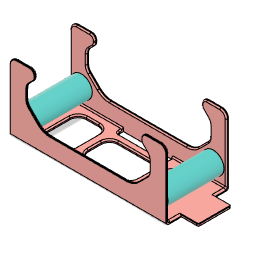
Spool Holder + Rollers D6 (Autodesk Fusion 360 design; units mm, degrees)
Autodesk Fusion 360 part; units mm, degrees
note: some values were not read from the file. Chosen so that the rebuilt part matches the saved one: which bodies a step acts on. Set by a fixed rule: which sketch regions a step uses.
sketch "Sketch1" plane through (0, 0, 0) normal (0, 1, 0) x (1, 0, 0) in component "Base"
  line L0 (-22.8106, -31.0965) -> (-3.5106, -30.609)
  line L1 (3.8, -23.1114) -> (3.8, 23.119)
  line L2 (40.5, -22.1842) -> (40.5, 22.1918)
  line L3 (13.7394, -30.1732) -> (33.1894, -29.6818)
  line L4 (13.7394, 30.1808) -> (33.1894, 29.6894)
  line L5 (-22.8106, 31.1041) -> (-3.5106, 30.6166)
  line L6 (-30.5, -23.5989) -> (-30.5, 23.6065)
  line L7 (6.05, -22.6756) -> (6.05, 22.6832)
  line L8 (95, 35) -> (-95, 35)
  line L9 (-95, 35) -> (-95, -35)
  line L10 (-95, -35) -> (95, -35)
  line L11 (95, -35) -> (95, 35)
  line L12 (95, 35) -> (-95, -35) construction
  line L13 (-95, 35) -> (95, -35) construction
  line L14 (-95, -35) -> (95, -35)
  line L15 (95, -35) -> (95, -38)
  line L16 (95, -38) -> (-95, -38)
  line L17 (-95, -38) -> (-95, -35)
  line L18 (-95, 35) -> (95, 35)
  line L19 (95, 35) -> (95, 38)
  line L20 (95, 38) -> (-95, 38)
  line L21 (-95, 38) -> (-95, 35)
  line L22 (0, -35) -> (0, 35) construction
  line L23 (-75, -25) -> (-40, -25)
  line L24 (-40, -25) -> (-40, 25)
  line L25 (-40, 25) -> (-75, 25)
  line L26 (-75, 25) -> (-75, -25)
  line L27 (40, -25) -> (75, -25)
  line L28 (75, -25) -> (75, 25)
  line L29 (75, 25) -> (40, 25)
  line L30 (40, 25) -> (40, -25)
  line L31 (-30, 18) -> (30, 18)
  line L32 (30, 18) -> (30, -18)
  line L33 (30, -18) -> (-30, -18)
  line L34 (-30, -18) -> (-30, 18)
  line L35 (-30, 38) -> (-30, 27)
  line L36 (30, 38) -> (30, 27)
  line L37 (-30, -27) -> (-30, -38)
  line L38 (30, -27) -> (30, -38)
  line L39 (-30, -27) -> (30, -27)
  line L40 (-30, 27) -> (30, 27)
  line L41 (95, 20) -> (114, 20)
  line L42 (116, 18) -> (116, -18)
  line L43 (114, -20) -> (95, -20)
  arc A0 (116, 18) -> (114, 20) centre (114, 18) ccw
  arc A1 (114, -20) -> (116, -18) centre (114, -18) ccw
  point P0 (-42.5, 38.6038)
  point P1 (-42.5, 36.7032)
  point P2 (52.5, 36.2038)
  point P3 (52.5, 34.3032)
  point P4 (52.5, -36.1962)
  point P5 (52.5, -34.2956)
  point P6 (-42.5, -36.6956)
  point P7 (-42.5, -38.5962)
  point P8 (52.5, 36.2038)
  point P9 (52.5, 34.3032)
  point P10 (52.5, -34.2956)
  point P11 (52.5, -36.1962)
  point P12 (-42.5, -38.5962)
  point P13 (-42.5, -36.6956)
  point P14 (-42.5, 36.7032)
  point P15 (-42.5, 38.6038)
  point P16 (0, -35)
  point P17 (0, 35)
  point P18 (0, 18)
  point P19 (-95, 0)
  point P20 (95, 0)
  point P21 (116, 20)
  dimension "d1" = 70
  dimension "d2" = 190
  dimension "d3" = 3
  dimension "d4" = 20
  dimension "d5" = 10
  dimension "d6" = 10
  dimension "d9" = 10
  dimension "d10" = 10
  dimension "d11" = 20
  dimension "d91" = 10
  dimension "d92" = 10
  dimension "d93" = 35
  dimension "d94" = 35
  dimension "d95" = 30
  dimension "d96" = 30
  dimension "d100" = 8
  dimension "d102" = 18
  dimension "d103" = 18
  dimension "d104" = 60
  dimension "d137" = 20
  dimension "d138" = 20
  dimension "d139" = 21
  dimension "d140" = 2
  dimension "d141" = 2
  constraint coincident P8 P2
  constraint coincident P9 P3
  constraint coincident P10 P5
  constraint coincident P11 P4
  constraint coincident P14 P1
  constraint coincident P15 P0
  constraint coincident P13 P6
  constraint coincident P12 P7
  constraint horizontal L8
  constraint perpendicular L8 L9
  constraint parallel L8 L10
  constraint parallel L9 L11
  constraint coincident L12 origin
  constraint coincident L13 origin
  constraint horizontal L14
  constraint vertical L15
  constraint horizontal L16
  constraint vertical L17
  constraint horizontal L18
  constraint vertical L19
  constraint horizontal L20
  constraint vertical L21
  constraint coincident L8.end L9.start
  constraint coincident L8.start L11.end
  constraint coincident L9.end L10.start
  constraint coincident L10.end L11.start
  constraint equal L17 L21
  constraint midpoint L14 P16
  constraint midpoint L8 P17
  constraint coincident P16 L22.start
  constraint coincident P17 L22.end
  constraint horizontal L23
  constraint vertical L24
  constraint horizontal L25
  constraint vertical L26
  constraint horizontal L27
  constraint vertical L28
  constraint horizontal L29
  constraint vertical L30
  constraint horizontal L31
  constraint vertical L32
  constraint horizontal L33
  constraint vertical L34
  constraint midpoint L31 P18
  constraint coincident L22 P18
  constraint vertical L35
  constraint vertical L36
  constraint perpendicular L16 L37
  constraint perpendicular L14 L38
  constraint coincident L20 L35.start
  constraint coincident L20 L36.start
  constraint coincident L16 L38.end
  constraint coincident L16 L37.end
  constraint horizontal L39
  constraint perpendicular L7 L40
  constraint coincident L37.start L39.start
  constraint coincident L38.start L39.end
  constraint coincident L35.end L40.start
  constraint coincident L36.end L40.end
  constraint collinear L35 L37
  constraint collinear L36 L38
  constraint equal L36 L38
  constraint midpoint L9 P19
  constraint midpoint L11 P20
  constraint horizontal L41
  constraint horizontal L43
  constraint vertical L42
  constraint coincident L11 L41.start
  constraint coincident L11 L43.end
  constraint coincident P21 L42
  constraint coincident P21 L41
  constraint tangent L42 A0
  constraint tangent L41 A0
  constraint tangent L42 A1
  constraint tangent L43 A1
  measures "d1" distance of L8.end L9.end
  measures "d2" distance of L8.start L8.end
  measures "d3" distance of L9.end L16.end
  measures "d4" distance of L9 L26
  measures "d5" distance of L14 L23
  measures "d6" distance of L8 L25
  measures "d9" distance of L18 L29
  measures "d10" distance of L10 L27
  measures "d11" distance of L11 L28
  measures "d91" distance of L24 L34
  measures "d92" distance of L30 L32
  measures "d93" distance of L24.end L25.end
  measures "d94" distance of L28 L30
  measures "d95" distance of P17 L35
  measures "d96" distance of P17 L36
  measures "d100" distance of L8 L40
  measures "d102" distance of origin L31
  measures "d103" distance of origin L33
  measures "d104" distance of L32 L34
  measures "d137" distance of P20 L43.end
  measures "d138" distance of P20 L41.start
  measures "d139" distance of L41.start P21
  measures "d140" radius of A0
  measures "d141" radius of A1
extrude "Extrude1" add sketch "Sketch1" along normal blind 100 contours L8 L18 L19 L20 L36 | L8 L18 L20 L35 L36 | L8 L18 L20 L21 L35 makes body 1 in component "Base"
extrude "Extrude2" add sketch "Sketch1" along normal blind 100 separate body contours L10 L14 L15 L16 L38 | L10 L14 L16 L17 L37 | L10 L14 L16 L37 L38 makes body 2 in component "Base"
extrude "Extrude3" add sketch "Sketch1" against normal blind 3 contours L8 L9 L10 L11 L14 L18 L35 L36 L37 L38 L39 L40 | L8 L18 L19 L20 L36 | L8 L18 L20 L35 L36 | L11 L41 L42 L43 A0 A1 | L8 L18 L20 L21 L35 | L10 L14 L15 L16 L38 | L10 L14 L16 L17 L37 | L10 L14 L16 L37 L38 bodies 1 2 in component "Base"
sketch "Sketch2" plane through (0, 0, -35) normal (0, 0, 1) x (1, 0, 0) in component "Base"
  circle A0 centre (-80, 20) radius 3.9
  circle A1 centre (-80, 20) radius 6
  line L0 (95, 0) -> (95, 100)
  line L1 (95, 100) -> (-95, 100)
  line L2 (-95, 100) -> (-95, 0)
  line L3 (-95, 0) -> (-30, 0)
  line L4 (0, 100) -> (0, 0) construction
  line L5 (-30, 0) -> (-30, -3)
  line L6 (-30, -3) -> (30, -3)
  line L7 (30, -3) -> (30, 0)
  line L8 (30, 0) -> (95, 0)
  line L9 (1.75, 0) -> (22.5, 0)
  line L10 (-55, 20) -> (55, 20)
  line L11 (55, 20) -> (75, 40)
  line L12 (-75, 40) -> (-55, 20)
  line L13 (65, 80) -> (95, 80)
  line L14 (65, 80) -> (65, 70)
  line L15 (65, 70) -> (75, 60)
  line L16 (75, 60) -> (75, 40)
  line L17 (-75, 40) -> (-75, 60)
  line L18 (-75, 60) -> (-65, 70)
  line L19 (-65, 70) -> (-65, 80)
  line L20 (-65, 80) -> (-95, 80)
  point P0 (-80, 20)
  point P1 (0, 20)
  point P2 (0, 80)
  dimension "d29" = 80
  dimension "d30" = 20
  dimension "d31" = 7.8
  dimension "d32" = 12
  dimension "d176" = 135
  dimension "d177" = 135
  dimension "d181" = 20
  dimension "d185" = 20
  dimension "d204" = 20
  dimension "d205" = 135
  dimension "d206" = 30
  dimension "d207" = 10
  dimension "d208" = 80
  dimension "d209" = 135
  constraint coincident P0 A0.centre
  constraint coincident L1 L4.start
  constraint coincident L4.end origin
  constraint horizontal L10
  constraint equal L11 L12
  constraint midpoint L10 P1
  constraint coincident L4 P1
  constraint coincident L4 P2
  constraint perpendicular L4 L9
  constraint horizontal L13
  constraint coincident L0 L13.end
  constraint vertical L16
  constraint coincident L13.start L14.start
  constraint vertical L14
  constraint coincident L2 L20.end
  constraint horizontal L20
  constraint vertical L19
  constraint vertical L17
  constraint equal L13 L20
  constraint equal L14 L19
  constraint equal L16 L17
  measures "d29" horizontal distance of P0 L4.end
  measures "d30" vertical distance of P0 L4.end
  measures "d31" diameter of A0
  measures "d32" diameter of A1
  measures "d176" angle of L10 L12
  measures "d177" angle of L10 L11
  measures "d181" distance of L8 L10
  measures "d185" vertical distance of L10.start L12.start
  measures "d204" distance of L0 L16
  measures "d205" angle of L14 L15
  measures "d206" distance of L13.start L13.end
  measures "d207" distance of L13.start L14.end
  measures "d208" distance of L8 L13
  measures "d209" angle of L18 L19
extrude "Extrude4" add sketch "Sketch2" along normal blind 6 separate body contours A0 makes body 3 in component "Base"
extrude "Extrude5" add sketch "Sketch2" along normal blind 2 contours A1 bodies 3 in component "Base"
extrude "Extrude9" cut sketch "Sketch2" along normal through all and the other way through all contours L0 L1 L2 L10 L11 L12 L13 L14 L15 L16 L17 L18 L19 L20 bodies 1 in component "Base"
sketch "Sketch3" plane through (0, 0, -29) normal (0, 0, 1) x (1, 0, 0) in component "Base"
  circle A0 centre (-80, 20) radius 3.9
  line L0 (-83.9, 20) -> (-76.1, 20)
  circle A1 centre (-80, 20) radius 3.9
  point P0 (-80, 20)
  point P1 (-80, 20)
  dimension "d37" = 7.8
  constraint coincident P0 A0.centre
  constraint horizontal L0
  constraint coincident P1 L0
  constraint coincident P1 P0
  constraint coincident L0.start A1
  constraint coincident L0.end A1
  measures "d37" diameter of A1
ref_plane "WorkPlane1" through (-80, 20, -29) normal (0, -0.707107, 0.707107) x (1, 0, 0) in component "Base"
split "Split1" by plane through (-80, 20, -29) normal (0, -0.707107, 0.707107) bodies 3 makes body 4 at (-83.0122, 17.5228, -30.5856) makes body 5 at (-80.4069, 14.0138, -33.6626) in component "Base"
delete_body "RemoveBody1" bodies 5 in component "Base"
delete_body "RemoveBody2" bodies 4 in component "Base"
mirror "Mirror1" about plane through (0, 0, 0) normal (1, 0, 0) of bodies 3 makes body 6 in component "Base"
mirror "Mirror2" about plane through (0, 0, 0) normal (0, 0, 1) of bodies 3 6 makes body 7 at (-83.318, 18.4237, 35) makes body 8 at (83.318, 18.4237, 35) in component "Base"
sketch "Sketch4" plane through (0, 0, -35) normal (0, 0, 1) x (1, 0, 0) in component "Base"
  circle A0 centre (0, 100) radius 100
  line L0 (0, 1.75) -> (0, 22.5)
  line L1 (-95, 100) -> (-95, 0)
  line L2 (95, 0) -> (95, 100)
  line L3 (30, 0) -> (95, 0)
  line L4 (95, 80) -> (65, 80)
  line L5 (75, 40) -> (55, 20)
  line L6 (55, 20) -> (-55, 20)
  line L7 (-55, 20) -> (-75, 40)
  line L8 (-95, 80) -> (-95, 0)
  line L9 (-95, 0) -> (-30, 0)
  line L10 (-30, 0) -> (-30, -3)
  line L11 (-30, -3) -> (30, -3)
  line L12 (30, -3) -> (30, 0)
  line L13 (30, 0) -> (95, 0)
  line L14 (95, 0) -> (95, 80)
  line L15 (-65, 80) -> (-95, 80)
  line L16 (65, 80) -> (65, 70)
  line L17 (65, 70) -> (75, 60)
  line L18 (75, 60) -> (75, 40)
  line L19 (-75, 40) -> (-75, 60)
  line L20 (-75, 60) -> (-65, 70)
  line L21 (-65, 70) -> (-65, 80)
  dimension "d44" = 200
  dimension "d45" = 100
  constraint coincident A0.centre L0
  measures "d44" diameter of A0
  measures "d45" distance of A0.centre origin
sketch "Sketch5" plane through (0, 0, -33) normal (0, 0, 1) x (1, 0, 0) in component "Base"
  line L0 (-84.4721, 16) -> (-75.5279, 16)
  arc A0 (-75.5279, 16) -> (-84.4721, 16) centre (-80, 20) ccw
  circle A1 centre (-80, 20) radius 3.9
  circle A2 centre (-80, 20) radius 4
  circle A3 centre (-80, 20) radius 5
  circle A4 centre (-80, 20) radius 11
  circle A5 centre (-80, 20) radius 10
  point P0 (-80, 20)
  point P1 (-80, 20)
  dimension "d48" = 8
  dimension "d49" = 10
  dimension "d50" = 22
  dimension "d51" = 20
  constraint coincident P1 P0
  constraint concentric A3 A5
  measures "d48" diameter of A2
  measures "d49" diameter of A3
  measures "d50" diameter of A4
  measures "d51" diameter of A5
extrude "Extrude6" add sketch "Sketch5" along normal blind 7 separate body contours L0 A3 | L0 A3 | A4 makes body 9 at (-69.0547, 18.9048, -28.3333) makes body 10 at (-75.0248, 20.4978, -28.3333) in component "Base"
extrude "Extrude8" add sketch "Sketch5" along normal blind 6 separate body contours L0 A0 A3 | A5 makes body 11 in component "Base"
move_face "OffsetFaces1" offset -1 1 faces at (-86.5028, 25.1815, -33) on bodies 11 in component "Base"
mirror "Mirror3" about plane through (0, 0, 0) normal (1, 0, 0) of bodies 9 10 11 makes body 12 at (69.0547, 18.9048, -28.3333) makes body 13 at (76.0199, 20.3983, -30.6667) makes body 14 at (86.5028, 25.1815, -32) in component "Base"
mirror "Mirror4" about plane through (0, 0, 0) normal (0, 0, 1) of bodies 9 13 12 14 11 10 makes body 15 at (-69.0547, 18.9048, 28.3333) makes body 16 at (-76.0199, 20.3983, 30.6667) makes body 17 at (-86.5028, 25.1815, 32) makes body 18 at (69.0547, 18.9048, 28.3333) makes body 19 at (76.0199, 20.3983, 30.6667) makes body 20 at (86.5028, 25.1815, 32) in component "Base"
fillet "Fillet6" radius 10 12 edges at (-75, -1.5, 25) (-75, -1.5, -25) (-40, -1.5, 25) (-40, -1.5, -25) (-30, -1.5, 18) (30, -1.5, 18) (-30, -1.5, -18) (30, -1.5, -18) (40, -1.5, 25) (75, -1.5, 25) (75, -1.5, -25) (40, -1.5, -25) on bodies 1 in component "Base"
fillet "Fillet6" radius 3 4 edges at (-30, -1.5, 27) (30, -1.5, 27) (-30, -1.5, -27) (30, -1.5, -27) on bodies 1 in component "Base"
chamfer "Chamfer2" distance 1.5 angle 45 4 edges at (-62.5, 0, -35) (62.5, 0, -35) (62.5, 0, 35) (-62.5, 0, 35) on bodies 1 in component "Base"
chamfer "Chamfer3" distance 2 angle 45 2 edges at (0, -3, 38) (0, -3, -38) on bodies 1 in component "Base"
fillet "Fillet4" radius 1.5 16 edges at (-75, 0, 0) (-72.0711, 0, -22.0711) (-57.5, 0, -25) (-42.9289, 0, -22.0711) (-40, 0, 0) (-42.9289, 0, 22.0711) (-57.5, 0, 25) (-72.0711, 0, 22.0711) (40, 0, 0) (42.9289, 0, -22.0711) (57.5, 0, -25) (72.0711, 0, -22.0711) (75, 0, 0) (72.0711, 0, 22.0711) (57.5, 0, 25) (42.9289, 0, 22.0711) on bodies 1 in component "Base"
fillet "Fillet4" radius 1.5 18 edges at (-27.0711, 0, -15.0711) (0, 0, -18) (27.0711, 0, -15.0711) (30, 0, 0) (27.0711, 0, 15.0711) (0, 0, 18) (-27.0711, 0, 15.0711) (-30, 0, 0) (30, 0, -31.75) (29.1213, 0, -27.8787) (0, 0, -27) (-29.1213, 0, -27.8787) (-30, 0, -31.75) (-30, 0, 31.75) (-29.1213, 0, 27.8787) (0, 0, 27) (29.1213, 0, 27.8787) (30, 0, 31.75) on bodies 1 in component "Base"
fillet "Fillet5" radius 2 7 edges at (95, 0, 26.75) (95, 0, -26.75) (95, 0.75, -34.25) (95, 0.75, 34.25) (-95, 0.75, -34.25) (-95, 0, 0) (-95, 0.75, 34.25) on bodies 1 in component "Base"
fillet "Fillet7" radius 10 8 edges at (-75, 40, 36.5) (-75, 60, 36.5) (75, 60, 36.5) (75, 40, 36.5) (-75, 60, -36.5) (-75, 40, -36.5) (75, 60, -36.5) (75, 40, -36.5) on bodies 1 in component "Base"
fillet "Fillet11" radius 6 8 edges at (-65, 70, 36.5) (-65, 80, 36.5) (65, 80, 36.5) (65, 70, 36.5) (-65, 80, -36.5) (-65, 70, -36.5) (65, 80, -36.5) (65, 70, -36.5) on bodies 1 in component "Base"
fillet "Fillet12" radius 8 4 edges at (-95, 80, 36.5) (-95, 80, -36.5) (95, 80, -36.5) (95, 80, 36.5) on bodies 1 in component "Base"
fillet "Fillet8" radius 20 4 edges at (-55, 20, 36.5) (-55, 20, -36.5) (55, 20, -36.5) (55, 20, 36.5) on bodies 1 in component "Base"
fillet "Fillet9" radius 0.5 32 edges at (95, 35.5, 38) (92.6569, 77.6569, 38) (79, 80, 38) (66.7574, 78.2426, 38) (65, 73.2426, 38) (65.4567, 70.1892, 38) (69.4142, 65.5858, 38) (74.2388, 59.6847, 38) (75, 50, 38) (74.2388, 40.3153, 38) (66.4645, 31.4645, 38) (54.3694, 21.5224, 38) (0, 20, 38) (-54.3694, 21.5224, 38) (-66.4645, 31.4645, 38) (-74.2388, 40.3153, 38) (-75, 50, 38) (-74.2388, 59.6847, 38) (-69.4142, 65.5858, 38) (-65.4567, 70.1892, 38) (-65, 73.2426, 38) (-66.7574, 78.2426, 38) (-79, 80, 38) (-92.6569, 77.6569, 38) (-95, 35.5, 38) (95, 35.5, -38) (92.6569, 77.6569, -38) (79, 80, -38) (66.7574, 78.2426, -38) (65, 73.2426, -38) (65.4567, 70.1892, -38) (69.4142, 65.5858, -38) on bodies 1 in component "Base"
fillet "Fillet9" radius 1.5 32 edges at (95, 35.3358, -35) (92.6569, 77.6569, -35) (79, 80, -35) (66.7574, 78.2426, -35) (65, 73.2426, -35) (65.4567, 70.1892, -35) (69.4142, 65.5858, -35) (-95, 35.3358, 35) (-92.6569, 77.6569, 35) (-79, 80, 35) (-66.7574, 78.2426, 35) (-65, 73.2426, 35) (-65.4567, 70.1892, 35) (-69.4142, 65.5858, 35) (-74.2388, 59.6847, 35) (-75, 50, 35) (-74.2388, 40.3153, 35) (-66.4645, 31.4645, 35) (-54.3694, 21.5224, 35) (0, 20, 35) (54.3694, 21.5224, 35) (66.4645, 31.4645, 35) (74.2388, 40.3153, 35) (75, 50, 35) (74.2388, 59.6847, 35) (69.4142, 65.5858, 35) (65.4567, 70.1892, 35) (65, 73.2426, 35) (66.7574, 78.2426, 35) (79, 80, 35) (92.6569, 77.6569, 35) (95, 35.3358, 35) on bodies 1 in component "Base"
chamfer "Chamfer4" distance 0.5 angle 45 10 edges at (104.5, -3, -20) (115.4142, -3, -19.4142) (116, -3, 0) (115.4142, -3, 19.4142) (104.5, -3, 20) (103.5, 0, -20) (115.4142, 0, -19.4142) (116, 0, 0) (115.4142, 0, 19.4142) (103.5, 0, 20) measured on face at (-88.3333, -3, -5) measured on face at (-88.3333, -3, -5) measured on face at (-88.3333, -3, -5) measured on face at (-88.3333, -3, -5) measured on face at (-88.3333, -3, -5) measured on face at (107.6667, -1.6667, -20) measured on face at (100.6667, 0, -6) measured on face at (116, -2, -6) measured on face at (100.6667, 0, -6) measured on face at (107.6667, -1.6667, 20) on bodies 1 in component "Base"
sketch "Sketch1 (2)" plane through (0, 0, -33) normal (0, 0, 1) x (1, 0, 0) in component "Roller"
  circle A0 centre (-80, 20) radius 11.1
  circle A1 centre (-80, 20) radius 13.1
  circle A2 centre (-80, 20) radius 9
  point P0 (-80, 20)
  point P1 (-80, 20)
  dimension "d63" = 22.2
  dimension "d64" = 26.2
  dimension "d65" = 18
  constraint coincident P0 A0.centre
  constraint coincident P1 P0
  measures "d63" diameter of A0
  measures "d64" diameter of A1
  measures "d65" diameter of A2
extrude "Extrude1'" add sketch "Sketch1 (2)" along normal blind 66 separate body contours A0 makes body 21 in component "Roller"
move_face "OffsetFaces1'" offset -7 1 faces at (-69.6413, 19.4485, 33) on bodies 21 in component "Roller"
move_face "OffsetFaces2" offset -7 1 faces at (-69.6413, 20.5515, -33) on bodies 21 in component "Roller"
extrude "Extrude2'" add sketch "Sketch1 (2)" along normal blind 67 contours A1 bodies 21 in component "Roller"
extrude "Extrude3'" add sketch "Sketch1 (2)" against normal blind 1 contours A1 bodies 21 in component "Roller"
chamfer "Chamfer1" distance 2.1 angle 30 1 edges at (-88.3909, 23.2545, 26) measured on face at (-69.6413, 20.5515, 26) on bodies 21 in component "Roller"
mirror "Mirror1'" about plane through (0, 0, 0) normal (1, 0, 0) of bodies 21 makes body 22 in component "Roller"
component "Base" placed x (1, 0, 0) y (0, 1, 0) z (0, 0, 1) at (0, 0, 0)
component "Roller" placed x (1, 0, 0) y (0, 1, 0) z (0, 0, 1) at (0, 0, 0)
equation "d1 = BaseInsideWidth"
equation "d2 = BaseLength"
equation "d3 = BaseWallThickness"
equation "d12 = BaseWallHeight"
equation "d14 = BaseWallHeight"
equation "d16 = -BaseWallThickness"
equation "BaseWallThickness = 3 mm"
equation "BearingHolderHeight = 20 mm"
equation "BearingHolderDistance = 80 mm"
equation "BearingHolderDiameter = 7.8 mm"
equation "d29 = BearingHolderDistance"
equation "d30 = BearingHolderHeight"
equation "d31 = BearingHolderDiameter"
equation "d37 = BearingHolderDiameter"
equation "BaseInsideWidth = 70 mm"
equation "BaseLength = 190 mm"
equation "BaseWallHeight = 100 mm"
equation "d66 = BaseInsideWidth - 4 mm"
equation "d70 = BaseInsideWidth + 1 mm - 2 mm - 2 mm"
